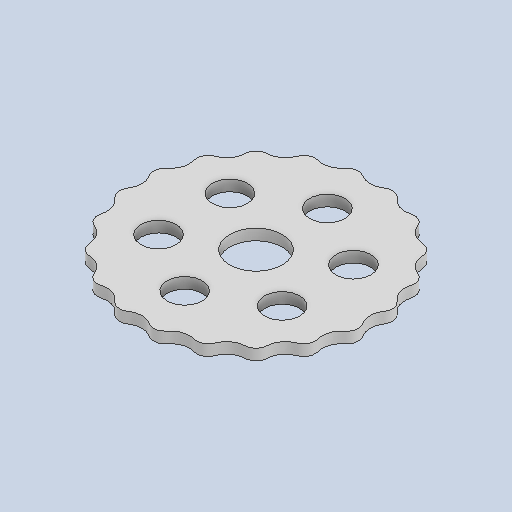
# Autodesk Inventor part: Epitrochoid
Saved by Autodesk Inventor 2023 (Build 270158000, 158)
## iProperties
Created: 2023-01-17
Part Number: Epitrochoid
Material: Generic
Document SubType Name: Modeling
Designer: caden
Density: 1 g/cm^3
Appearance: Default
Description: 3D Print
Author: caden
Autodesk Inventor part; units mm, degrees
ref_plane "YZ Plane" through (0, 0, 0) normal (1, 0, 0) x (0, 1, 0)
ref_plane "XZ Plane" through (0, 0, 0) normal (0, 1, 0) x (-1, 0, 0)
ref_plane "XY Plane" through (0, 0, 0) normal (0, 0, 1) x (1, 0, 0)
sketch "Sketch2" plane through (0, 0, 0) normal (0, 1, 0) x (-1, 0, 0)
  spline S0 degree 5 poles (52, 0) (51.9967, -1.037) (52.1807, -2.0631) (52.4953, -3.0783) (53.1947, -4.2876) (53.8569, -5.5176) (54.0094, -5.8481) (54.2651, -6.561) (54.3843, -7.3093) (54.4073, -7.703) (54.3774, -8.4952) (54.1962, -9.2674) (54.0674, -9.6461) (53.7537, -10.3344) (53.3177, -10.951) (53.0871, -11.2235) (52.2124, -12.1066) (51.2628, -12.9126) (50.6877, -13.6017) (49.5394, -15.3441) (49.0221, -17.3736) (48.9233, -18.5824) (49.1679, -20.1198) (49.4762, -21.6389) (49.5353, -22.0139) (49.5922, -22.7776) (49.5055, -23.5396) (49.4248, -23.9181) (49.1862, -24.6724) (48.808, -25.3668) (48.5804, -25.7021) (48.0929, -26.2837) (47.5061, -26.764) (47.2122, -26.9629) (46.2484, -27.5049) (45.2189, -27.9135) (44.5566, -28.272) (42.8439, -29.4158) (41.5598, -31.0444) (40.9511, -32.2435) (40.585, -33.9071) (40.4032, -35.5896) (40.3539, -35.9915) (40.2001, -36.7615) (39.9055, -37.4896) (39.7303, -37.8264) (39.3022, -38.4869) (38.7564, -39.0535) (38.4451, -39.3187) (37.8161, -39.7525) (37.1173, -40.0617) (36.7789, -40.1747) (35.8144, -40.4087) (34.823, -40.4806) (34.1951, -40.5636) (32.2225, -40.9778) (30.4292, -41.939) (29.3454, -42.8815) (28.314, -44.3924) (27.5591, -46.0411) (27.381, -46.4476) (27.0108, -47.1775) (26.5114, -47.8253) (26.2582, -48.0979) (25.6739, -48.6171) (25.0023, -49.0161) (24.6299, -49.1898) (23.902, -49.4433) (23.1392, -49.5563) (22.7782, -49.5747) (21.8732, -49.5429) (20.9877, -49.348) (20.4594, -49.2337) (18.5301, -48.9293) (16.5646, -49.1067) (15.168, -49.5895) (13.5565, -50.6511) (12.2315, -52.0271) (11.9005, -52.4026) (11.3113, -53.0421) (10.6151, -53.5616) (10.3046, -53.7533) (9.6091, -54.0952) (8.8622, -54.3004) (8.4565, -54.3688) (7.6806, -54.4209) (6.9083, -54.3257) (6.5491, -54.2458) (5.7458, -53.99) (5.0033, -53.5893) (4.597, -53.3485) (2.9589, -52.4483) (1.1577, -51.8845) (-0.3059, -51.8117) (-2.2758, -52.1812) (-4.0619, -53.0451) (-4.5659, -53.3311) (-5.3729, -53.8192) (-6.2518, -54.1579) (-6.5966, -54.2581) (-7.3511, -54.4011) (-8.1188, -54.4009) (-8.5269, -54.359) (-9.295, -54.2026) (-10.0197, -53.9029) (-10.3514, -53.727) (-11.0211, -53.2872) (-11.5972, -52.7303) (-11.8819, -52.4158) (-13.0673, -51.1132) (-14.437, -49.984) (-15.708, -49.3956) (-17.7131, -48.9456) (-19.7446, -49.106) (-20.42, -49.2163) (-21.4304, -49.4723) (-22.4665, -49.5704) (-22.8219, -49.5743) (-23.5807, -49.5118) (-24.3148, -49.3092) (-24.6945, -49.1615) (-25.3981, -48.805) (-26.021, -48.3205) (-26.2994, -48.0575) (-26.8096, -47.4734) (-27.2017, -46.805) (-27.3726, -46.4524) (-28.0418, -44.966) (-28.8308, -43.5296) (-29.7103, -42.5868) (-31.3885, -41.349) (-33.3628, -40.714) (-34.1608, -40.5439) (-35.3258, -40.4665) (-36.4721, -40.2566) (-36.8152, -40.1645) (-37.5254, -39.904) (-38.1754, -39.5153) (-38.4988, -39.2747) (-39.0852, -38.7423) (-39.559, -38.1074) (-39.7612, -37.7736) (-40.0906, -37.0866) (-40.2856, -36.3514) (-40.3507, -35.9854) (-40.5295, -34.5154) (-40.7259, -33.0423) (-41.1306, -31.9722) (-42.1655, -30.147) (-43.7434, -28.7706) (-44.5465, -28.2287) (-45.7557, -27.7148) (-46.9293, -27.1308) (-47.2386, -26.9473) (-47.8528, -26.5077) (-48.3749, -25.9601) (-48.6194, -25.6468) (-49.0443, -24.9769) (-49.3333, -24.2382) (-49.4412, -23.8563) (-49.5743, -23.1113) (-49.5657, -22.3561) (-49.5309, -21.9975) (-49.3075, -20.6909) (-49.0131, -19.3953) (-48.9858, -18.4116) (-49.1917, -16.3267) (-50.0792, -14.4252) (-50.7057, -13.4859) (-51.7757, -12.4764) (-52.8473, -11.4758) (-53.1031, -11.2081) (-53.5805, -10.6168) (-53.9395, -9.9455) (-54.0894, -9.5845) (-54.3213, -8.8268) (-54.404, -8.0389) (-54.4067, -7.6364) (-54.3361, -6.8826) (-54.1263, -6.1561) (-53.9978, -5.8247) (-53.4846, -4.7642) (-52.8568, -3.7646) (-52.5245, -3.0046) (-51.8928, -1.0267) (-51.9281, 1.0602) (-52.1802, 2.3118) (-52.8809, 3.7782) (-53.6827, 5.1822) (-53.8653, 5.5264) (-54.172, 6.2362) (-54.3412, 6.9914) (-54.3888, 7.3721) (-54.4112, 8.1613) (-54.2826, 8.9399) (-54.1773, 9.3331) (-53.9069, 10.0445) (-53.509, 10.6929) (-53.2959, 10.9771) (-52.5977, 11.7628) (-51.7882, 12.4358) (-51.2964, 12.9274) (-49.9798, 14.488) (-49.1809, 16.3851) (-48.9205, 17.7527) (-49.0393, 19.5122) (-49.3954, 21.2258) (-49.4809, 21.6377) (-49.5893, 22.4287) (-49.5484, 23.2259) (-49.494, 23.5981) (-49.3071, 24.3603) (-48.9788, 25.0728) (-48.7714, 25.4264) (-48.318, 26.0452) (-47.7571, 26.5687) (-47.4728, 26.7872) (-46.6736, 27.3003) (-45.7963, 27.6674) (-45.2617, 27.912) (-43.5123, 28.8598) (-42.0627, 30.2519) (-41.2712, 31.4806) (-40.6838, 33.2647) (-40.4543, 35.1109) (-40.4105, 35.576) (-40.2958, 36.4073) (-40.0289, 37.2022) (-39.8807, 37.5398) (-39.5006, 38.2194) (-38.9993, 38.8149) (-38.7043, 39.1015) (-38.0977, 39.5821) (-37.4113, 39.9406) (-37.0738, 40.0774) (-36.2379, 40.3338) (-35.3683, 40.4323) (-34.8639, 40.4803) (-32.9651, 40.7501) (-31.1567, 41.4457) (-29.9497, 42.3001) (-28.6666, 43.7908) (-27.7883, 45.5278) (-27.5739, 46.0163) (-27.2113, 46.84) (-26.7059, 47.5834) (-26.4773, 47.8641) (-25.9347, 48.413) (-25.2993, 48.8506) (-24.9389, 49.0482) (-24.2205, 49.3537) (-23.4569, 49.5178) (-23.0881, 49.5607) (-22.2667, 49.5808) (-21.4554, 49.4477) (-21.0178, 49.3513) (-19.23, 48.9937) (-17.3909, 48.9519) (-15.9875, 49.2851) (-14.1676, 50.1845) (-12.6837, 51.5416) (-12.2558, 51.9954) (-11.6195, 52.7472) (-10.8676, 53.3812) (-10.5763, 53.5876) (-9.9132, 53.9687) (-9.1907, 54.2197) (-8.7926, 54.314) (-8.0134, 54.4191) (-7.228, 54.3738) (-6.8536, 54.3161) (-6.0899, 54.1228) (-5.3758, 53.7908) (-5.0198, 53.5921) (-3.5411, 52.7444) (-1.9644, 52.0672) (-0.6247, 51.8622) (1.444, 51.963) (3.3679, 52.6889) (4.0344, 53.0123) (4.9604, 53.5989) (5.9566, 54.0516) (6.2907, 54.1711) (7.0255, 54.3605) (7.7833, 54.4099) (8.1886, 54.3952) (8.972, 54.2896) (9.7211, 54.0361) (10.0734, 53.8777) (10.7403, 53.4966) (11.3236, 52.9985) (11.5925, 52.728) (12.6485, 51.5742) (13.7644, 50.4682) (14.8167, 49.8379) (16.7692, 49.0832) (18.8527, 49.0063) (19.7335, 49.0713) (20.9297, 49.3649) (22.1453, 49.5476) (22.5011, 49.5726) (23.2563, 49.5597) (23.997, 49.4057) (24.3792, 49.2855) (25.1087, 48.9751) (25.7655, 48.5308) (26.0685, 48.2799) (26.6026, 47.7411) (27.0258, 47.1131) (27.2039, 46.7939) (27.8106, 45.5206) (28.3948, 44.2322) (29.0365, 43.373) (30.5163, 41.8848) (32.4065, 40.9748) (33.3973, 40.6541) (34.7743, 40.5106) (36.1425, 40.3247) (36.4986, 40.2515) (37.2242, 40.0373) (37.8981, 39.6905) (38.2296, 39.4764) (38.8509, 38.9835) (39.3665, 38.3809) (39.5955, 38.0534) (39.9652, 37.3936) (40.2047, 36.6776) (40.2883, 36.3301) (40.487, 35.0888) (40.5848, 33.8328) (40.8139, 32.9494) (41.5667, 31.0013) (42.9214, 29.4028) (43.8359, 28.6283) (45.2138, 27.9363) (46.61, 27.2971) (46.9459, 27.1241) (47.5947, 26.7192) (48.1572, 26.1995) (48.4152, 25.9101) (48.8826, 25.2715) (49.2191, 24.5556) (49.3547, 24.1742) (49.5355, 23.4376) (49.5759, 22.6808) (49.5627, 22.3263) (49.4293, 21.2165) (49.1519, 20.1316) (49.0553, 19.3719) (48.989, 17.3103) (49.5715, 15.3173) (50.187, 14.134) (51.3165, 12.8766) (52.5614, 11.749) (52.8547, 11.4739) (53.3835, 10.8964) (53.7955, 10.2302) (53.964, 9.8892) (54.2436, 9.153) (54.3779, 8.3773) (54.4075, 7.9698) (54.3859, 7.2065) (54.2218, 6.4608) (54.1136, 6.1212) (53.7277, 5.1968) (53.1992, 4.3446) (52.8913, 3.7799) (52.6322, 3.184) (52.4269, 2.5736) knots 0 0 0 0 0 0 0.014369 0.014369 0.014369 0.019405 0.019405 0.019405 0.024846 0.024846 0.024846 0.030369 0.030369 0.030369 0.035299 0.035299 0.035299 0.047636 0.047636 0.047636 0.063941 0.063941 0.063941 0.069193 0.069193 0.069193 0.07454 0.07454 0.07454 0.080129 0.080129 0.080129 0.085031 0.085031 0.085031 0.09547 0.09547 0.09547 0.113377 0.113377 0.113377 0.118993 0.118993 0.118993 0.124238 0.124238 0.124238 0.129874 0.129874 0.129874 0.134806 0.134806 0.134806 0.143626 0.143626 0.143626 0.162628 0.162628 0.162628 0.168801 0.168801 0.168801 0.173943 0.173943 0.173943 0.179606 0.179606 0.179606 0.184604 0.184604 0.184604 0.192142 0.192142 0.192142 0.211635 0.211635 0.211635 0.218612 0.218612 0.218612 0.223656 0.223656 0.223656 0.229326 0.229326 0.229326 0.234413 0.234413 0.234413 0.24099 0.24099 0.24099 0.260338 0.260338 0.260338 0.268417 0.268417 0.268417 0.273381 0.273381 0.273381 0.279035 0.279035 0.279035 0.284223 0.284223 0.284223 0.290115 0.290115 0.290115 0.308691 0.308691 0.308691 0.318206 0.318206 0.318206 0.323119 0.323119 0.323119 0.328736 0.328736 0.328736 0.334028 0.334028 0.334028 0.339457 0.339457 0.339457 0.356693 0.356693 0.356693 0.367964 0.367964 0.367964 0.372871 0.372871 0.372871 0.378432 0.378432 0.378432 0.383822 0.383822 0.383822 0.38896 0.38896 0.38896 0.404418 0.404418 0.404418 0.41767 0.41767 0.41767 0.422637 0.422637 0.422637 0.428125 0.428125 0.428125 0.433604 0.433604 0.433604 0.43858 0.43858 0.43858 0.452028 0.452028 0.452028 0.467299 0.467299 0.467299 0.472418 0.472418 0.472418 0.477817 0.477817 0.477817 0.483372 0.483372 0.483372 0.488281 0.488281 0.488281 0.49973 0.49973 0.49973 0.516814 0.516814 0.516814 0.522212 0.522212 0.522212 0.527513 0.527513 0.527513 0.533125 0.533125 0.533125 0.538035 0.538035 0.538035 0.547699 0.547699 0.547699 0.566173 0.566173 0.566173 0.572016 0.572016 0.572016 0.577213 0.577213 0.577213 0.582865 0.582865 0.582865 0.587822 0.587822 0.587822 0.596018 0.596018 0.596018 0.615321 0.615321 0.615321 0.621825 0.621825 0.621825 0.626922 0.626922 0.626922 0.632591 0.632591 0.632591 0.637627 0.637627 0.637627 0.64469 0.64469 0.64469 0.664197 0.664197 0.664197 0.671635 0.671635 0.671635 0.67664 0.67664 0.67664 0.682305 0.682305 0.682305 0.687437 0.687437 0.687437 0.693672 0.693672 0.693672 0.712745 0.712745 0.712745 0.721434 0.721434 0.721434 0.726371 0.726371 0.726371 0.732011 0.732011 0.732011 0.737246 0.737246 0.737246 0.742903 0.742903 0.742903 0.760936 0.760936 0.760936 0.771211 0.771211 0.771211 0.776115 0.776115 0.776115 0.781709 0.781709 0.781709 0.787046 0.787046 0.787046 0.792324 0.792324 0.792324 0.808799 0.808799 0.808799 0.820949 0.820949 0.820949 0.825873 0.825873 0.825873 0.831403 0.831403 0.831403 0.836836 0.836836 0.836836 0.841886 0.841886 0.841886 0.856449 0.856449 0.856449 0.870623 0.870623 0.870623 0.875646 0.875646 0.875646 0.881096 0.881096 0.881096 0.886611 0.886611 0.886611 0.891546 0.891546 0.891546 0.904077 0.904077 0.904077 0.920205 0.920205 0.920205 0.925433 0.925433 0.925433 0.930789 0.930789 0.930789 0.936372 0.936372 0.936372 0.941274 0.941274 0.941274 0.951882 0.951882 0.951882 0.969656 0.969656 0.969656 0.975232 0.975232 0.975232 0.980486 0.980486 0.980486 0.986119 0.986119 0.986119 0.991046 0.991046 0.991046 1 1 1 1 1 1
  arc A0 (52.4269, 2.5736) -> (52, 0) centre (59.9711, 0) ccw
  point P0 (0, 0)
  constraints: 2 point on circle, 1 centre point, 4 other
extrude "Extrusion2" add sketch "Sketch2" along normal blind 5
sketch "Sketch3" plane through (0, 5, 0) normal (0, 1, 0) x (1, 0, 0)
  circle A0 centre (0, 0) radius 12
  circle A1 centre (0, 0) radius 32.5 construction
  circle A2 centre (0, 32.5) radius 8
  circle A3 centre (-28.1458, 16.25) radius 8
  circle A4 centre (-28.1458, -16.25) radius 8
  circle A5 centre (0, -32.5) radius 8
  circle A6 centre (28.1458, -16.25) radius 8
  circle A7 centre (28.1458, 16.25) radius 8
  circle A8 centre (0, 32.5) radius 7.25 construction
  circle A9 centre (0, 32.5) radius 11 construction
  dimension "d12" = 65
  dimension "d10" = 24
  dimension "d11" = 16
  dimension "d15" = 360
  dimension "d20" = 14.5
  dimension "d21" = 22
  constraints: 9 centre point, 4 coincident, 1 vertical alignment, 15 other
  measures "d10" diameter of A0
  measures "d11" diameter of A2
  measures "d20" diameter of A8
  measures "d21" diameter of A9
extrude "Extrusion3" cut sketch "Sketch3" against normal through all
equation "curve S0 of \"Sketch2\": x = (60*cos(t))-(6.5*cos(t+atan(sin((1-21)*t)/((60/(1.5*21))-cos((1-21)*t)))))-(1.5*cos(21*t)); y = (-60*sin(t))+(6.5*sin(t+atan(sin((1-21)*t)/((60/(1.5*21))-cos((1-21)*t)))))+("
body "Solid2"
